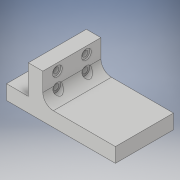
# Autodesk Inventor part: Test Stand
Saved by Autodesk Inventor 2019 (Build 230136000, 136)
## iProperties
Created: 2020-04-08
Part Number: Test Stand
Material: Generic
Document SubType Name: Modeling
Designer: isaac
Density: 1 g/cm^3
Appearance: Default
Author: isaac
Autodesk Inventor part; units mm, degrees
ref_plane "YZ Plane" through (0, 0, 0) normal (1, 0, 0) x (0, 1, 0)
ref_plane "XZ Plane" through (0, 0, 0) normal (0, 1, 0) x (-1, 0, 0)
ref_plane "XY Plane" through (0, 0, 0) normal (0, 0, 1) x (1, 0, 0)
sketch "Sketch1" plane through (0, 0, 0) normal (0, 0, 1) x (1, 0, 0)
  line L0 (0, 0) -> (10, 0)
  line L1 (10, 0) -> (10, 20)
  line L2 (10, 20) -> (0, 20)
  line L3 (0, 20) -> (0, 0)
  line L4 (10, 0) -> (-15, 0)
  line L5 (-15, 0) -> (-15, -10)
  line L6 (-15, -10) -> (10, -10)
  line L7 (10, -10) -> (10, 0)
  line L8 (10, -10) -> (60, -10)
  line L9 (60, -10) -> (60, 0)
  line L10 (60, 0) -> (10, 0)
  line L11 (10, 0) -> (10, -10)
  dimension "d0" = 10
  dimension "d1" = 20
  dimension "d2" = 25
  dimension "d3" = 10
  dimension "d4" = 50
  constraints: 24 end point, 6 parallel, 3 horizontal, 3 perpendicular, 1 point on line
  measures "d0" distance of L2.end L1.end
  measures "d1" distance of L1.end L0.end
  measures "d2" distance of L6.end L5.end
  measures "d3" distance of L5.end L4.end
  measures "d4" distance of L10.end L9.end
extrude "Extrusion1" add sketch "Sketch1" along normal blind 40
sketch "Sketch2" plane through (10, 20, 40) normal (1, 0, 0) x (0, 0, -1)
  line L0 (40, 0) -> (0, 0) construction
  line L1 (40, -20) -> (0, -20) construction
  line L2 (0, -20) -> (0, 0) construction
  line L3 (0, 0) -> (40, 0) construction
  line L4 (40, 0) -> (40, -20) construction
  line L5 (40, 0) -> (40, -20) construction
  line L6 (0, 0) -> (40, -20) construction
  line L7 (0, 0) -> (0, -20) construction
  line L8 (40, 0) -> (0, -20) construction
  line L9 (10, -15) -> (30, -15) construction
  line L10 (30, -15) -> (30, -5) construction
  line L11 (30, -5) -> (10, -5) construction
  line L12 (10, -5) -> (10, -15) construction
  line L13 (10, -15) -> (30, -5) construction
  line L14 (30, -15) -> (10, -5) construction
  point P0 (20, -10)
  dimension "d9" = 20
  constraints: 24 end point, 4 coincident, 4 parallel, 3 midpoint, 2 horizontal, 2 perpendicular, 1 point on line
  measures "d9" distance of L11.end L10.end
hole "Hole1" at (10, 15, 30) at (10, 15, 10) at (10, 5, 10) at (10, 5, 30) direction (-1, 0, 0) diameter 3.9 end through all counterbore diameter 6.75 counterbore depth 1
fillet "Fillet3" radius 7.25 1 edges at (10, 0, 20)
body "Solid1"
